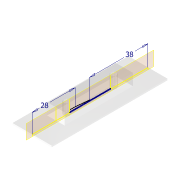
# Autodesk Inventor part: 00_chip
Saved by Autodesk Inventor 2022 (Build 260153000, 153)
## iProperties
Created: 2022-02-01
Part Number: 00_chip
Material: Generisch
Document SubType Name: Modeling
Designer: diederichbenedict
Density: 1 g/cm^3
Appearance: Polycarbonat - klar
Author: diederichbenedict
Autodesk Inventor part; units mm, degrees
ref_plane "YZ Plane" through (0, 0, 0) normal (1, 0, 0) x (0, 1, 0)
ref_plane "XZ Plane" through (0, 0, 0) normal (0, 1, 0) x (-1, 0, 0)
ref_plane "XY Plane" through (0, 0, 0) normal (0, 0, 1) x (1, 0, 0)
sketch "Skizze1" plane through (0, 0, 0) normal (0, 1, 0) x (-1, 0, 0)
  line L0 (0, 0) -> (-25.4, 0)
  line L1 (-25.4, 0) -> (-25.4, 75.5)
  line L2 (-25.4, 75.5) -> (0, 75.5)
  line L3 (0, 75.5) -> (0, 0)
  dimension "d0" = 25.4
  dimension "d1" = 75.5
  constraints: 8 end point, 2 parallel, 1 horizontal, 1 perpendicular
  measures "d0" distance of L1.end L2.end
  measures "d1" distance between parallel lines of L0 L2
extrude "Extrusion1" add sketch "Skizze1" along normal blind 1
sketch "Skizze2" plane through (0, 1, 0) normal (0, 1, 0) x (1, 0, 0)
  line L0 (0, -75.5) -> (25.4, -75.5) projected
  line L1 (25.4, -75.5) -> (25.4, 0) projected
  line L2 (25.4, 0) -> (0, 0) projected
  line L3 (0, 0) -> (0, -75.5) projected
  line L4 (7, -60) -> (18.4, -60)
  line L5 (18.4, -60) -> (18.4, -15.5)
  line L6 (18.4, -15.5) -> (7, -15.5)
  line L7 (7, -15.5) -> (7, -60)
  dimension "d4" = 7
  dimension "d5" = 7
  dimension "d6" = 15.5
  dimension "d7" = 15.5
  constraints: 8 end point, 2 parallel, 1 horizontal, 1 perpendicular
  measures "d4" distance between parallel lines of L7 L3
  measures "d5" distance between parallel lines of L1 L5
  measures "d6" distance between parallel lines of L2 L6
  measures "d7" distance between parallel lines of L0 L4
extrude "Extrusion2" add sketch "Skizze2" along normal blind 7.5 contours L7 L6 L5 L4
sketch "Skizze3" plane through (0, 8.5, 0) normal (0, 1, 0) x (1, 0, 0)
  line L0 (18.4, -60) -> (18.4, -15.5) projected
  line L1 (18.4, -15.5) -> (7, -15.5) projected
  line L2 (7, -15.5) -> (7, -60) projected
  line L3 (7, -60) -> (18.4, -60) projected
  circle A0 centre (12.7, -53) radius 1.7919
  circle A1 centre (12.7, -22.5) radius 1.7997
  point P0 (0, 0)
  dimension "d10" = 7
  dimension "d11" = 7
  constraints: 2 centre point
  measures "d10" distance from line of L3 A0.centre
  measures "d11" distance from line of A1.centre L1
extrude "Extrusion3" cut sketch "Skizze3" against normal up to surface (7.5 mm away) contours A0 | A1
ref_plane "Arbeitsebene1" through (12.7, 0, 75.5) normal (1, 0, 0) x (0, 0, -1)
sketch "Skizze5" plane through (12.7, 1, 60) normal (1, 0, 0) x (0, 0, -1)
  line L0 (8.3796, 0.5) -> (36.1482, 0.5) projected
  line L1 (-15.5, 0) -> (60, 0) projected
  line L2 (8.7919, 7.5) -> (8.7919, 0) projected
  line L3 (8.7919, 1.6191) -> (12.5, 1.6191)
  line L4 (12.5, 1.6191) -> (22, 0.7063)
  line L5 (22, 0.7063) -> (22, 0.5)
  line L6 (36.1103, 0.5) -> (8.3796, 0.5) projected
  line L7 (0, 0) -> (0, 7.5) projected
  line L8 (-15.5, -1) -> (-15.5, 0) projected
  line L9 (60, -1) -> (60, 0) projected
  line L10 (35.7003, 7.5) -> (35.7003, 0) projected
  line L11 (44.5, 0) -> (0, 0) projected
  line L12 (35.7003, 0.5) -> (8.7919, 0.5)
  line L13 (8.7919, 0.5) -> (8.7919, 0)
  line L14 (8.7919, 0) -> (35.7003, 0)
  line L15 (35.7003, 0) -> (35.7003, 0.5)
  line L16 (8.7919, 1.6191) -> (8.7919, 0.5)
  point P0 (35.7003, 0.5)
  point P1 (22, 0.5)
  dimension "d17" = 28
  dimension "d18" = 38
  constraints: 16 end point, 3 point on line, 2 horizontal, 2 parallel, 1 collinear, 1 perpendicular, 1 vertical, 4 other
  measures "d17" distance from line of L8 L3.end
  measures "d18" distance from line of L9 L4.end
extrude "Extrusion5" cut sketch "Skizze5" along normal mid plane 2
sketch "Skizze6" plane through (0, 0, 0) normal (0, -1, 0) x (1, 0, 0)
  line L0 (13.7, 47.5) -> (11.7, 47.5) projected
  line L1 (11.7, 38) -> (13.7, 38) projected
  circle A0 centre (12.7, 40.1939) radius 1.0539
  point P0 (0, 0)
  constraints: 1 centre point
extrude "Extrusion6" cut sketch "Skizze6" against normal blind 0.1
equation "\"d12\" = d11"
